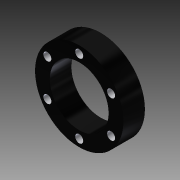
# Autodesk Inventor part: 550 Sprocket Spacer (am-0651)
Saved by Autodesk Inventor 2013 (Build 170138000, 138)
## iProperties
Created: 2013-08-13
Part Number: 550 Sprocket Spacer (am-0651)
Material: PC/ABS Plastic
Document SubType Name: Modeling
Designer: Creo
Density: 1 g/cm^3
Author: Creo
Autodesk Inventor part; units mm, degrees
ref_plane "YZ Plane" through (0, 0, 0) normal (1, 0, 0) x (0, 1, 0)
ref_plane "XZ Plane" through (0, 0, 0) normal (0, 1, 0) x (-1, 0, 0)
ref_plane "XY Plane" through (0, 0, 0) normal (0, 0, 1) x (1, 0, 0)
sketch "Sketch1" plane through (0, 0, 0) normal (0, 0, 1) x (1, 0, 0)
  circle A0 centre (0, 0) radius 28.575
  circle A1 centre (0, 0) radius 19.05
  dimension "d0" = 57.15
  dimension "d8" = 38.1
  constraints: 2 centre point, 1 coincident
  measures "d0" diameter of A0
  measures "d8" diameter of A1
sketch "Sketch2" plane through (0, 0, 0) normal (0, 0, 1) x (1, 0, 0)
  circle A0 centre (0, 0) radius 23.8125
  circle A1 centre (0, 23.8125) radius 2.5908
  circle A2 centre (-20.6222, 11.9063) radius 2.5908
  circle A3 centre (-20.6222, -11.9062) radius 2.5908
  circle A4 centre (0, -23.8125) radius 2.5908
  circle A5 centre (20.6222, -11.9063) radius 2.5908
  circle A6 centre (20.6222, 11.9062) radius 2.5908
  dimension "d15" = 47.625
  dimension "d16" = 5.1816
  dimension "d19" = 360
  constraints: 6 centre point, 1 coincident, 1 vertical alignment, 15 other
  measures "d16" diameter of A1
extrude "Extrusion1" add sketch "Sketch1" along normal blind 13.97
extrude "Extrusion2" cut sketch "Sketch2" along normal blind 13.97 contours A6 A0 | A0 A6 | A5 A0 | A0 A5 | A1 A0 | A0 A1 | A4 A0 | A0 A4 | A2 A0 | A0 A2 | A3 A0 | A0 A3
body "Solid1"
